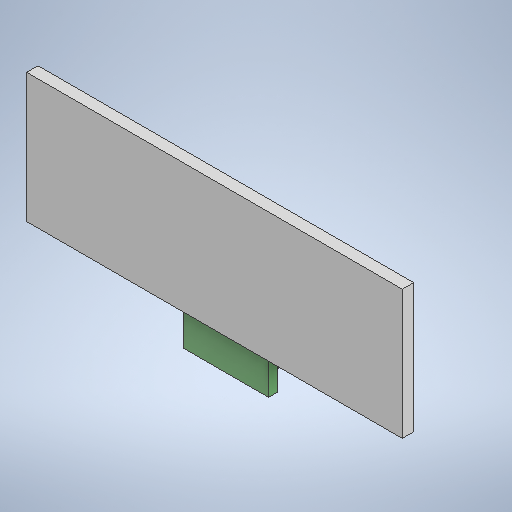
# Autodesk Inventor part: AE-AQM1602A
Saved by Autodesk Inventor 2025.3 (Build 293356000, 356)
## iProperties
Created: 2025-05-29
Part Number: AE-AQM1602A
Material: 一般
Document SubType Name: Modeling
Designer: yamashita1
Density: 1 g/cm^3
Appearance: 既定
Author: yamashita1
Autodesk Inventor part; units mm, degrees
ref_plane "YZ Plane" through (0, 0, 0) normal (1, 0, 0) x (0, 1, 0)
ref_plane "XZ Plane" through (0, 0, 0) normal (0, 1, 0) x (-1, 0, 0)
ref_plane "XY Plane" through (0, 0, 0) normal (0, 0, 1) x (1, 0, 0)
sketch "スケッチ1" plane through (0, 0, 0) normal (0, 0, 1) x (1, 0, 0)
  line L0 (-33, 22.7) -> (33, 22.7)
  line L1 (33, 22.7) -> (33, 0)
  line L2 (33, 0) -> (-33, 0)
  line L3 (-33, 0) -> (-33, 22.7)
  point P0 (0, 0)
  point P1 (0, 0)
  dimension "d0" = 66
  dimension "d1" = 22.7
  constraints: 8 end point, 2 parallel, 1 coincident, 1 horizontal, 1 midpoint, 1 perpendicular
  measures "d0" distance of L1.end L2.end
  measures "d1" distance of L0.end L1.end
extrude "押し出し1" add sketch "スケッチ1" along normal blind 2
sketch "スケッチ3" plane through (0, 0, 0) normal (0, 0, -1) x (-1, 0, 0)
  line L0 (-7.5, 4) -> (7.5, 4)
  line L1 (7.5, 4) -> (7.5, -7.5)
  line L2 (7.5, -7.5) -> (-7.5, -7.5)
  line L3 (-7.5, -7.5) -> (-7.5, 4)
  line L4 (33, 0) -> (-33, 0) projected
  point P0 (0, 0)
  point P1 (0, 4)
  point P2 (0, 0)
  dimension "d4" = 15
  dimension "d5" = 11.5
  dimension "d6" = 4
  constraints: 8 end point, 2 midpoint, 2 parallel, 1 horizontal, 1 perpendicular, 1 vertical alignment
  measures "d4" distance of L1.end L2.end
  measures "d5" distance of L0.end L1.end
  measures "d6" distance between parallel lines of L0 L4
extrude "押し出し2" add sketch "スケッチ3" along normal blind 1.6
sketch "スケッチ4" plane through (0, 0, -1.6) normal (0, 0, -1) x (-1, 0, 0)
  line L0 (-5.08, -3.81) -> (5.08, -3.81)
  line L1 (5.08, -3.81) -> (5.08, -6.35)
  line L2 (5.08, -6.35) -> (-5.08, -6.35)
  line L3 (-5.08, -6.35) -> (-5.08, -3.81)
  point P0 (0, 0)
  point P1 (0, -3.81)
  point P2 (5.08, -5.08)
  dimension "d9" = 10.16
  dimension "d10" = 2.54
  dimension "d11" = 5.08
  constraints: 8 end point, 2 midpoint, 2 parallel, 1 horizontal, 1 perpendicular, 1 vertical alignment
  measures "d9" distance of L1.end L2.end
  measures "d10" distance of L0.end L1.end
  measures "d11" horizontal distance of point (0, 0) point (5.08, -5.08)
extrude "押し出し3" add sketch "スケッチ4" along normal blind 11
